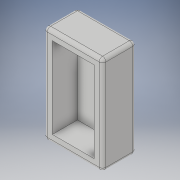
# Autodesk Inventor part: Inner Block
Saved by Autodesk Inventor 2017 (Build 210142000, 142)
## iProperties
Created: 2017-10-25
Part Number: Inner Block
Material: Generic
Document SubType Name: Modeling
Designer: Tripl_000
Density: 1 g/cm^3
Appearance: Default
Author: Tripl_000
Autodesk Inventor part; units mm, degrees
ref_plane "YZ Plane" through (0, 0, 0) normal (1, 0, 0) x (0, 1, 0)
ref_plane "XZ Plane" through (0, 0, 0) normal (0, 1, 0) x (-1, 0, 0)
ref_plane "XY Plane" through (0, 0, 0) normal (0, 0, 1) x (1, 0, 0)
sketch "Sketch1" plane through (0, 0, 0) normal (0, 0, 1) x (1, 0, 0)
  line L0 (-17.5, 29.25) -> (17.5, 29.25)
  line L1 (17.5, 29.25) -> (17.5, -29.25)
  line L2 (17.5, -29.25) -> (-17.5, -29.25)
  line L3 (-17.5, -29.25) -> (-17.5, 29.25)
  line L4 (-17.5, 29.25) -> (17.5, -29.25) construction
  line L5 (17.5, 29.25) -> (-17.5, -29.25) construction
  point P0 (0, 0)
  dimension "d0" = 35
  dimension "d1" = 58.5
  constraints: 12 end point, 2 midpoint, 2 parallel, 1 horizontal, 1 perpendicular
  measures "d0" distance of L0.start L0.end
  measures "d1" distance of L2.end L0.start
extrude "Extrusion1" add sketch "Sketch1" along normal blind 20
sketch "Sketch2" plane through (0, 0, 20) normal (0, 0, 1) x (1, 0, 0)
  line L0 (-12.5, 24.25) -> (12.5, 24.25)
  line L1 (12.5, 24.25) -> (12.5, -24.25)
  line L2 (12.5, -24.25) -> (-12.5, -24.25)
  line L3 (-12.5, -24.25) -> (-12.5, 24.25)
  line L4 (-12.5, 24.25) -> (12.5, -24.25) construction
  line L5 (12.5, 24.25) -> (-12.5, -24.25) construction
  point P0 (0, 0)
  dimension "d4" = 25
  dimension "d5" = 48.5
  constraints: 12 end point, 2 midpoint, 2 parallel, 1 horizontal, 1 perpendicular
  measures "d4" distance of L0.start L0.end
  measures "d5" distance of L2.end L0.start
extrude "Extrusion2" cut sketch "Sketch2" against normal blind 15
fillet "Fillet1" radius 2 12 edges at (17.5, 29.25, 10) (-17.5, 29.25, 10) (17.5, -29.25, 10) (-17.5, -29.25, 10) (0, 29.25, 20) (17.5, 0, 20) (0, -29.25, 20) (-17.5, 0, 20) (17.5, 0, 0) (0, 29.25, 0) (-17.5, 0, 0) (0, -29.25, 0)
body "Solid1"
